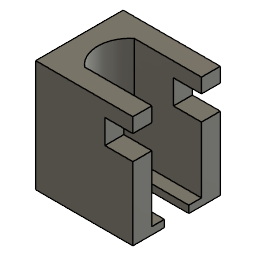
Motor Mount (Autodesk Fusion 360 design; units mm, degrees)
part number: 2026-05-27-11-24-24-823
Autodesk Fusion 360 part; units mm, degrees
sketch "Sketch1" plane through (0, 0, 0) normal (0, 1, 0) x (1, 0, 0)
  line L0 (-10, -9) -> (10, -9)
  line L1 (10, -9) -> (10, 9)
  line L2 (10, 9) -> (-10, 9)
  line L3 (-10, 9) -> (-10, -9)
  line L4 (-10, 0) -> (10, 0) construction
  line L5 (0, 9) -> (0, -9) construction
  dimension "d1" = 18
  dimension "d2" = 20
  constraint horizontal L0
  constraint vertical L1
  constraint horizontal L2
  constraint vertical L3
  constraint midpoint L3 L4.start
  constraint midpoint L1 L4.end
  constraint midpoint L2 L5.start
  constraint midpoint L0 L5.end
  constraint coincident origin L4
  constraint coincident origin L5
  measures "d1" distance of L0.start L2.end
  measures "d2" distance of L1.end L2.end
extrude "Extrude1" add sketch "Sketch1" along normal blind 23
sketch "Sketch2" plane through (0, 0, 0) normal (0, -1, 0) x (1, 0, 0)
  line L0 (-10, 9) -> (-10, -9)
  line L1 (-10, -9) -> (10, -9)
  line L2 (10, -9) -> (10, 9)
  line L3 (10, 9) -> (-10, 9)
  line L4 (10, 2.5) -> (0, 2.5)
  line L5 (10, -2.5) -> (0, -2.5)
  arc A0 (0, 2.5) -> (0, -2.5) centre (0, 0) ccw
  line L6 (10, 2.5) -> (10, -2.5)
  dimension "d5" = 2.5
  constraint coincident L2 L4.start
  constraint perpendicular L2 L4
  constraint coincident L2 L5.start
  constraint perpendicular L2 L5
  constraint tangent L4 A0
  constraint tangent L5 A0
  constraint coincident A0.centre origin
  measures "d5" radius of A0
extrude "Extrude2" cut sketch "Sketch2" against normal blind 1.5 contours L2 L4 L5 A0 L6
sketch "Sketch3" plane through (0, 1.5, 0) normal (0, -1, 0) x (1, 0, 0)
  arc A0 (0, 2.5) -> (0, -2.5) centre (0, 0) ccw
  line L0 (0, -2.5) -> (10, -2.5)
  line L1 (10, -2.5) -> (10, 2.5)
  line L2 (10, 2.5) -> (0, 2.5)
  line L3 (10, 5.1) -> (-6.2, 5.1)
  line L4 (-6.2, 5.1) -> (-6.2, -5.1)
  line L5 (-6.2, -5.1) -> (10, -5.1)
  line L6 (10, -5.1) -> (10, 5.1)
  line L7 (-6.2, 0) -> (10, 0) construction
  dimension "d9" = 10.2
  dimension "d10" = 6.2
  constraint horizontal L3
  constraint vertical L4
  constraint horizontal L5
  constraint vertical L6
  constraint coincident L0.end L6
  constraint midpoint L4 L7.start
  constraint midpoint L6 L7.end
  constraint coincident A0.centre L7
  measures "d9" distance of L3.end L4.end
  measures "d10" distance of A0.centre L4
extrude "Extrude3" cut sketch "Sketch3" against normal blind 9.5
sketch "Sketch4" plane through (0, 11, 0) normal (0, -1, 0) x (1, 0, 0)
  line L0 (10, -5.1) -> (10, 5.1)
  line L1 (10, 5.1) -> (-6.2, 5.1)
  line L2 (-6.2, 5.1) -> (-6.2, -5.1)
  line L3 (-6.2, -5.1) -> (10, -5.1)
  arc A0 (-3.8, 5.1) -> (-3.8, -5.1) centre (0.4187, 0) ccw
  line L4 (-3.8, 5.1) -> (10, 5.1)
  line L5 (10, -5.1) -> (-3.8, -5.1)
  dimension "d13" = 2.4
  constraint coincident L3 A0.end
  constraint coincident L1 A0.start
  constraint vertical A0.start A0.end
  constraint tangent L2 A0
  constraint coincident L0.end L1.start
  constraint coincident L0.start L3.end
  measures "d13" distance of L2 A0.start
extrude "Extrude4" cut sketch "Sketch4" against normal through all contours L0 L1 L3 A0 L4 L5
sketch "Sketch6" plane through (0, 23, 0) normal (0, 1, 0) x (-1, 0, 0)
  line L0 (3.8, -5.1) -> (-10, -5.1)
  line L1 (-10, -5.1) -> (-10, -9)
  line L2 (-10, -9) -> (10, -9)
  line L3 (10, -9) -> (10, 9)
  line L4 (10, 9) -> (-10, 9)
  line L5 (-10, 9) -> (-10, 5.1)
  line L6 (-10, 5.1) -> (3.8, 5.1)
  arc A0 (3.8, -5.1) -> (3.8, 5.1) centre (-0.4187, 0) ccw
  line L7 (-10, 9) -> (-4.25, 9)
  line L8 (-4.25, 9) -> (-4.25, 5.1)
  line L9 (-4.25, 5.1) -> (-10, 5.1)
  line L10 (-10, 5.1) -> (-10, 9)
  line L11 (-2.5, 0) -> (-20, 0)
  line L12 (-4.25, -9) -> (-4.25, -5.1)
  line L13 (-10, -9) -> (-4.25, -9)
  line L14 (-10, -5.1) -> (-10, -9)
  line L15 (-4.25, -5.1) -> (-10, -5.1)
  dimension "d17" = 5.75
  constraint horizontal L7
  constraint vertical L8
  constraint horizontal L9
  constraint vertical L10
  constraint coincident L6 L8.end
  constraint coincident L4.end L5.start
  constraint symmetric L4.end L11 L1.end
  constraint symmetric L7.end L11 L12.start
  constraint symmetric L8.end L11 L12.end
  constraint symmetric L5.end L11 L0.end
  measures "d17" distance of L4.end L7.end
extrude "Extrude5" cut sketch "Sketch6" against normal blind 5 from surface at -3 contours L0 L1 L2 L12 L13 L14 L15 | L4 L5 L6 L7 L8 L9 L10
